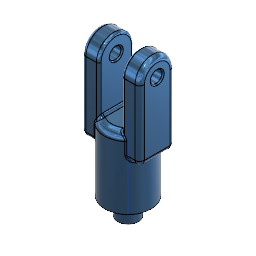
Link 0 (Autodesk Fusion 360 design; units mm, degrees)
Autodesk Fusion 360 part; units mm, degrees
sketch "Sketch2" plane through (0, 0, 0) normal (0, 0, 1) x (1, 0, 0)
  line L0 (-45, 75) -> (45, 75)
  line L1 (-45, 75) -> (45, 75)
  line L2 (-45, 150) -> (45, 150)
  line L3 (0, 75) -> (0, 450)
  line L4 (0, 450) -> (100, 450)
  line L5 (100, 450) -> (100, 150)
  line L6 (100, 150) -> (45, 150)
  line L7 (45, 150) -> (45, 75)
  dimension "d1" = 100
  dimension "d2" = 300
  constraint midpoint L0 L3.start
  constraint perpendicular L0 L3
  constraint perpendicular L3 L4
  constraint perpendicular L4 L5
  constraint perpendicular L5 L6
  constraint coincident L0.end L1.end
  constraint vertical L7
  constraint coincident L2.end L6.end
  measures "d1" distance of L3.end L4.end
  measures "d2" distance of L4.end L5.end
revolve "Revolve1" add sketch "Sketch2" angle 360 about axis through (0, 75, 0) along (0, 1, 0) makes body 1
ref_plane "WorkPlane1" through (50, 0, 0) normal (1, 0, 0) x (0, 1, 0)
sketch "Sketch1" plane through (50, 0, 0) normal (1, 0, 0) x (0, 0, -1)
  line L0 (-75, 650) -> (-75, 350)
  arc A0 (-75, 350) -> (75, 350) centre (0, 350) ccw
  line L1 (75, 350) -> (75, 650)
  arc A1 (75, 650) -> (-75, 650) centre (0, 650) ccw
  line L2 (0, 650) -> (0, 350) construction
  line L3 (-75, 350) -> (75, 350)
  line L4 (-100, 450) -> (100, 450)
  circle A2 centre (0, 650) radius 25
  dimension "d17" = 100
  dimension "d18" = 50
  dimension "d19" = 200
  dimension "d20" = 75
  constraint tangent L0 A0
  constraint tangent A0 L1
  constraint parallel L0 L1
  constraint tangent L1 A1
  constraint tangent L0 A1
  constraint vertical L2
  constraint perpendicular L1 L3
  constraint vertical origin A0.centre
  constraint concentric A1 A2
  measures "d17" distance of L3 L4
  measures "d18" diameter of A2
  measures "d19" distance of L4 A1.centre
  measures "d20" radius of A1
extrude "Extrude1" add sketch "Sketch1" along normal blind 75 separate body contours L0 L1 A1 L4 | L0 L1 L3 L4 makes body 2
fillet "Fillet1" radius 30 1 edges at (-93.2327, 450, -36.1615) on bodies 1
fillet "Fillet2" radius 20 3 edges at (125, 500, -75) (125, 725, 0) (125, 500, 75) on bodies 2
fillet "Fillet3" radius 20 5 edges at (77.5, 350, 75) (119.1421, 350, 69.1421) (125, 350, 0) (119.1421, 350, -69.1421) (77.5, 350, -75) on bodies 2
fillet "Fillet4" radius 10 6 edges at (50, 350, 0) (50, 355.8579, -69.1421) (50, 510, -75) (50, 725, 0) (50, 510, 75) (50, 355.8579, 69.1421) on bodies 2
chamfer "Chamfer1" distance 5 angle 45 2 edges at (50, 659.0404, 23.3082) (125, 659.0404, 23.3082) on bodies 2
mirror "Mirror1" about plane through (0, 0, 0) normal (1, 0, 0) of bodies 2 makes body 3
combine "Combine1" operation add target body 1 tool bodies 2
combine "Combine2" operation add target body 1 tool bodies 3
fillet "Fillet5" radius 10 24 edges at (50, 450, 0) (50, 449.4189, -57.0712) (53.5781, 442.1049, -72.6655) (64.4901, 427.9989, -75) (66.1438, 395, -75) (72.7701, 355.3269, -68.5883) (100, 350, 0) (72.7701, 355.3269, 68.5883) (66.1438, 395, 75) (64.4901, 427.9989, 75) (53.5633, 442.1221, 72.6531) (50, 449.4189, 57.0712) (-66.1438, 395, 75) (-72.7701, 355.3269, 68.5883) (-100, 350, 0) (-72.7701, 355.3269, -68.5883) (-66.1438, 395, -75) (-64.4901, 427.9989, -75) (-53.5633, 442.1221, -72.6531) (-50, 449.4189, -57.0712) (-50, 450, 0) (-50, 449.4189, 57.0712) (-53.5781, 442.1049, 72.6655) (-64.4901, 427.9989, 75) on bodies 1
